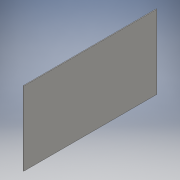
# Autodesk Inventor part: TMP
Saved by Autodesk Inventor 2016 (Build 200138000, 138)
## iProperties
Created: 2016-01-13
Part Number: TMP
Material: Generic
Document SubType Name: Modeling
Designer: Douglas
Density: 1 g/cm^3
Appearance: Default
Author: Douglas
Autodesk Inventor part; units mm, degrees
ref_plane "YZ Plane" through (0, 0, 0) normal (1, 0, 0) x (0, 1, 0)
ref_plane "XZ Plane" through (0, 0, 0) normal (0, 1, 0) x (-1, 0, 0)
ref_plane "XY Plane" through (0, 0, 0) normal (0, 0, 1) x (1, 0, 0)
sketch "Sketch1" plane through (0, 0, 0) normal (1, 0, 0) x (0, 1, 0)
  line L0 (0, 0) -> (330.2, 0)
  line L1 (330.2, 0) -> (330.2, -596.9)
  line L2 (330.2, -596.9) -> (0, -596.9)
  line L3 (0, -596.9) -> (0, 0)
  dimension "d0" = 330.2
  dimension "d1" = 596.9
  constraints: 8 end point, 2 parallel, 1 horizontal, 1 perpendicular
  measures "d0" distance of L1.end L2.end
  measures "d1" distance of L0.end L1.end
extrude "Extrusion1" add sketch "Sketch1" along normal blind 3.175
body "Solid1"
